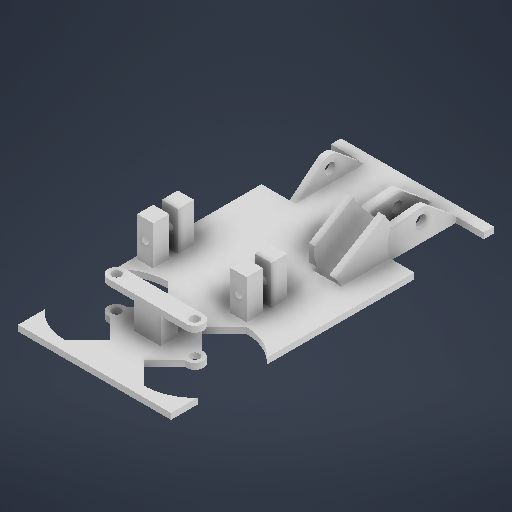
# Autodesk Inventor part: Рама
Saved by Autodesk Inventor 2026.2 (Build 302298000, 298)
## iProperties
Created: 2026-02-19
Part Number: Рама
Material: Типовые
Document SubType Name: Modeling
Designer: Leonid
Density: 1 g/cm^3
Appearance: По умолчанию
Author: Leonid
Autodesk Inventor part; units mm, degrees
ref_plane "XZ Plane" through (0, 0, 0) normal (0, 1, 0) x (-1, 0, 0)
ref_plane "XY Plane" through (0, 0, 0) normal (0, 0, 1) x (1, 0, 0)
sketch "Эскиз1" plane through (0, 0, 0) normal (0, 1, 0) x (-1, 0, 0)
  line L0 (-22.5, -47.5) -> (22.5, -47.5)
  line L1 (22.5, -47.5) -> (22.5, 14.5)
  line L2 (22.5, 47.5) -> (-22.5, 47.5)
  line L3 (-22.5, 47.5) -> (-22.5, 44.5)
  line L4 (-22.5, -47.5) -> (22.5, 47.5) construction
  line L5 (22.5, -47.5) -> (-22.5, 47.5) construction
  line L6 (22.5, 29.5) -> (-22.5, 29.5) construction
  line L7 (-22.5, 44.5) -> (-22.5, 14.5)
  line L8 (-22.5, 14.5) -> (-22.5, -47.5)
  line L9 (22.5, 14.5) -> (22.5, 44.5)
  line L10 (22.5, 44.5) -> (22.5, 47.5)
  circle A0 centre (11.5, 29.5) radius 1.325
  line L11 (22.5, 44.5) -> (5, 44.5)
  line L12 (-22.5, 44.5) -> (-5, 44.5)
  arc A1 (11.5, 27) -> (11.5, 32) centre (11.5, 29.5) ccw
  line L13 (11.5, 32) -> (5, 32)
  circle A2 centre (-11.5, 29.5) radius 1.325
  arc A3 (-11.5, 32) -> (-11.5, 27) centre (-11.5, 29.5) ccw
  line L14 (-11.5, 32) -> (-5, 32)
  line L15 (11.5, 27) -> (-11.5, 27)
  line L16 (22.5, 14.5) -> (-22.5, 14.5)
  line L17 (5, 32) -> (5, 44.5)
  line L18 (-5, 32) -> (-5, 44.5)
  line L19 (-11.5, 44.5) -> (-5, 38)
  line L20 (-11.5, 44.5) -> (-2.3076, 44.5) construction
  line L21 (11.5, 44.5) -> (5, 38)
  line L22 (11.5, 44.5) -> (20.6924, 44.5) construction
  line L23 (5, 38) -> (11, 32)
  line L24 (-5, 38) -> (-11, 32)
  arc A4 (-11.5, 44.5) -> (-22.5, 39.698) centre (-11.5, 29.5) ccw
  arc A5 (22.5, 39.698) -> (11.5, 44.5) centre (11.5, 29.5) ccw
  arc A6 (-22.5, 19.302) -> (-11.5, 14.5) centre (-11.5, 29.5) ccw
  arc A7 (11.5, 14.5) -> (22.5, 19.302) centre (11.5, 29.5) ccw
  line L25 (-11.5, 44.5) -> (-11.5, 14.5) construction
  line L26 (11.5, 44.5) -> (11.5, 14.5) construction
  line L27 (-11, 27) -> (-5, 21)
  line L28 (-11, 27) -> (-2.5147, 27) construction
  line L29 (-5, 21) -> (-11.5, 14.5)
  line L30 (11.5, 14.5) -> (5, 21)
  line L31 (11.5, 14.5) -> (20.6924, 14.5) construction
  line L32 (5, 21) -> (11, 27)
  line L33 (-5.8, 8.55) -> (-10.55, 8.55)
  line L34 (-10.55, 8.55) -> (-10.55, 13.3)
  line L35 (-10.55, 13.3) -> (-5.8, 13.3)
  line L36 (-5.8, 13.3) -> (-5.8, 8.55)
  line L37 (16.95, 8.55) -> (21.7, 8.55)
  line L38 (21.7, 8.55) -> (21.7, 13.3)
  line L39 (21.7, 13.3) -> (16.95, 13.3)
  line L40 (16.95, 13.3) -> (16.95, 8.55)
  line L41 (-5.8, 1.3) -> (-10.55, 1.3)
  line L42 (-10.55, 1.3) -> (-10.55, 6.05)
  line L43 (-10.55, 6.05) -> (-5.8, 6.05)
  line L44 (-5.8, 6.05) -> (-5.8, 1.3)
  line L45 (16.95, 1.3) -> (21.7, 1.3)
  line L46 (21.7, 1.3) -> (21.7, 6.05)
  line L47 (21.7, 6.05) -> (16.95, 6.05)
  line L48 (16.95, 6.05) -> (16.95, 1.3)
  line L49 (22.5, -44.5) -> (-22.5, -44.5)
  line L50 (-22.5, -24.104) -> (-14.25, -24.104)
  line L51 (-14.25, -24.104) -> (-14.25, -44.5)
  line L52 (22.5, -24.104) -> (14.25, -24.104)
  line L53 (14.25, -24.104) -> (14.25, -44.5)
  line L54 (-12.5, -25.63) -> (-7, -25.63)
  line L55 (-7, -25.63) -> (-7, -42.974)
  line L56 (-7, -42.974) -> (-12.5, -42.974)
  line L57 (-12.5, -42.974) -> (-12.5, -25.63)
  line L58 (-12.5, -34.302) -> (-14.25, -34.302) construction
  line L59 (-7.8, 13.3) -> (16.95, 13.3)
  line L60 (16.95, 13.3) -> (16.95, -11.2)
  line L61 (16.95, -11.2) -> (-7.8, -11.2)
  line L62 (-7.8, -11.2) -> (-7.8, 13.3)
  line L63 (-4, 27) -> (4, 27)
  line L64 (4, 27) -> (4, 32)
  line L65 (4, 32) -> (-4, 32)
  line L66 (-4, 32) -> (-4, 27)
  line L67 (-4, 27) -> (4, 32) construction
  line L68 (4, 27) -> (-4, 32) construction
  point P0 (0, 0)
  point P1 (13.75, 44.5)
  point P2 (-12.5, -44.5)
  point P3 (-7.8, 1.3)
  point P4 (16.95, 1.3)
  point P5 (-7.8, 8.55)
  point P6 (-7.8, 6.05)
  point P7 (0, 29.5)
  point P8 (-4, 27)
  point P9 (4, 27)
  dimension "d0" = 45
  dimension "d6" = 3
  dimension "d7" = 2.65
  dimension "d8" = 11
  dimension "d14" = 2.65
  dimension "d15" = 11
  dimension "d16" = 2.5
  dimension "d19" = 10
  dimension "d20" = 12.5
  dimension "d22" = 95
  dimension "d23" = 12.5
  dimension "d25" = 23
  dimension "d26" = 45
  dimension "d27" = 135
  dimension "d29" = 23
  dimension "d30" = 45
  dimension "d31" = 135
  dimension "d37" = 0.5
  dimension "d38" = 32.25
  dimension "d39" = 22.75
  dimension "d40" = 4.75
  dimension "d42" = 5.95
  dimension "d43" = 32.25
  dimension "d44" = 22.75
  dimension "d45" = 4.75
  dimension "d46" = 2.5
  dimension "d60" = 20.3961
  dimension "d61" = 3
  dimension "d62" = 20.396
  dimension "d63" = 8.25
  dimension "d70" = 5.55
  dimension "d71" = 1.75
  dimension "d72" = 5.5
  dimension "d73" = 17.344
  dimension "d101" = 24.5
  dimension "d102" = 2
  dimension "d120" = 8
  constraints: 138 end point, 31 point on line, 23 perpendicular, 22 parallel, 17 horizontal, 12 point on circle, 11 equal length, 10 midpoint, 8 centre point, 6 coincident, 6 collinear, 6 tangent, 1 vertical
  measures "d0" distance of L2.end L2.start
  measures "d6" distance of L9.end L2.start
  measures "d7" diameter of A0
  measures "d8" distance from line of A0.centre L9
  measures "d14" diameter of A2
  measures "d15" distance from line of L7 A2.centre
  measures "d16" radius of A3
  measures "d19" distance between parallel lines of L18 L17
  measures "d20" distance between parallel lines of L16 L15
  measures "d22" distance between parallel lines of L0 L2
  measures "d23" vertical distance of L3.end L14.start
  measures "d25" distance of A2.centre A0.centre
  measures "d26" angle of L19 L20
  measures "d27" angle of L21 L22
  measures "d29" distance of L19.start L21.start
  measures "d30" angle of L27 L28
  measures "d31" angle of L31 L30
  measures "d37" distance of L15.start L32.end
  measures "d38" distance between parallel lines of L34 L38
  measures "d39" distance between parallel lines of L36 L40
  measures "d40" distance between parallel lines of L35 L33
  measures "d42" distance from line of L25.end L33
  measures "d43" distance between parallel lines of L42 L46
  measures "d44" distance between parallel lines of L44 L48
  measures "d45" distance between parallel lines of L43 L41
  measures "d46" distance between parallel lines of L33 L43
  measures "d60" distance of A6.start A4.end
  measures "d61" distance between parallel lines of L0 L49
  measures "d62" distance of L49.end L50.start
  measures "d63" distance of L50.start L50.end
  measures "d70" distance between parallel lines of L1 L40
  measures "d71" distance between parallel lines of L51 L57
  measures "d72" distance between parallel lines of L57 L55
  measures "d73" distance between parallel lines of L56 L54
  measures "d101" distance between parallel lines of L59 L61
  measures "d102" distance between parallel lines of L44 L62
  measures "d120" distance between parallel lines of L64 L66
extrude "Выдавливание1" add sketch "Эскиз1" along normal blind 1.75 contours L8 L49 L1 L0 | L8 L16 L1 L52 L53 L49 L51 L50 | L7 A6 L16 | L16 A7 L9 | L29 L27 L15 L32 L30 L16 | L7 L12 A4 | A5 L11 L9 | L3 L2 L10 L11 L17 L13 A1 L15 L64 L65 L66 A3 L14 L18 L12 | L12 L18 L19 | L21 L17 L11 | L18 L14 L24 | L66 L65 L64 L15 | L23 L13 L17 | L36 L59 L40 L60 L48 L61 L62 L41 L44 L43 L33 | L33 L62 L35 L36 | L33 L34 L35 L62 | L62 L41 L42 L43 | L43 L44 L41 L62 | L39 L38 L37 L40 | L47 L46 L45 L48
extrude "Выдавливание3" add sketch "Эскиз1" along normal blind 13.25 contours L33 L62 L35 L36 | L33 L34 L35 L62 | L62 L41 L42 L43 | L43 L44 L41 L62 | L39 L38 L37 L40 | L47 L46 L45 L48
sketch "Эскиз3" plane through (10.55, 1.75, 1.3) normal (0, 0, -1) x (-1, 0, 0)
  line L0 (-11.95, 0) -> (33.05, 0) projected
  line L1 (0, 0) -> (0, 11.5) projected
  point P0 (10.55, -1.75)
  point P1 (2.375, 5.95)
  point P2 (29.875, 5.95)
  dimension "d49" = 27.5
  dimension "d50" = 5.95
  dimension "d51" = 2.375
  dimension "d52" = 5.95
  measures "d49" distance of point (29.875, 5.95) point (2.375, 5.95)
  measures "d50" distance from line of L0 point (2.375, 5.95)
  measures "d51" distance from line of L1 point (2.375, 5.95)
  measures "d52" distance from line of L0 point (29.875, 5.95)
hole "Отверстие1" at (8.175, 7.7, 1.3) at (-19.325, 7.7, 1.3) direction (0, 0, 1) diameter 2.1 end through all
sketch "Эскиз4" plane through (14.25, 0, -24.104) normal (1, 0, 0) x (0, 0, -1)
  line L0 (0, 1.75) -> (20.396, 1.75) projected
  circle A0 centre (10.198, 5.6) radius 1.575
  line L1 (10.198, 5.6) -> (10.198, 1.75) construction
  arc A1 (12.4201, 8.3041) -> (7.9759, 8.3041) centre (10.198, 5.6) ccw
  line L2 (0, 1.75) -> (7.9759, 8.3041)
  line L3 (12.4201, 8.3041) -> (20.396, 1.75)
  point P0 (-24.104, 0)
  dimension "d64" = 3.15
  dimension "d65" = 3.85
  dimension "d66" = 3.5
  constraints: 6 end point, 2 centre point, 2 point on circle, 2 tangent, 1 coincident, 1 midpoint, 1 vertical
  measures "d64" diameter of A0
  measures "d65" distance of L1.start L1.end
  measures "d66" radius of A1
extrude "Выдавливание4" add sketch "Эскиз4" against normal blind 1.75
mirror "Зеркальное отражение1" about plane through (0, 0, 0) normal (1, 0, 0) of "Выдавливание4"
ref_plane "РабПлоскость2" through (9.85, 0, 0) normal (1, 0, 0) x (0, 1, 0)
sketch "Эскиз5" plane through (9.85, 0, 0) normal (1, 0, 0) x (0, 1, 0)
  circle A0 centre (5.6, -34.302) radius 1.575 projected
  line L0 (5.6, -34.302) -> (5.6, -24.814)
  line L1 (1.75, -24.104) -> (1.75, -25.63) projected
  arc A1 (14.3322, -38.0128) -> (5.6, -24.814) centre (5.6, -34.302) ccw
  line L2 (6.8478, -6.6784) -> (15.6371, -21.2299)
  line L3 (15.6371, -21.2299) -> (8.7893, -25.3661)
  line L4 (8.7893, -25.3661) -> (0, -10.8145)
  line L5 (0, -10.8145) -> (6.8478, -6.6784)
  line L6 (16.0736, -20.9662) -> (8.3528, -25.6297)
  line L7 (8.3528, -25.6297) -> (14.557, -35.9014)
  line L8 (14.557, -35.9014) -> (22.2779, -31.2379)
  line L9 (22.2779, -31.2379) -> (16.0736, -20.9662)
  line L10 (22.2779, -31.2379) -> (8.3528, -25.6297) construction
  line L11 (5.6, -34.302) -> (19.1758, -26.1021) construction
  line L12 (0, 19.302) -> (0, -24.104) projected
  line L13 (13.4972, -22.5225) -> (4.7079, -7.9709)
  line L14 (1.75, 30.825) -> (1.75, 28.175) projected
  line L15 (1.75, 30.825) -> (1.75, 28.175) projected
  line L16 (1.75, 13.3) -> (1.75, 8.55) projected
  line L17 (1.75, 8.55) -> (1.75, 13.3) projected
  line L18 (1.75, 8.55) -> (1.75, 13.3) projected
  line L19 (1.75, 13.3) -> (1.75, 8.55) projected
  line L20 (1.75, 1.3) -> (1.75, 6.05) projected
  line L21 (1.75, 6.05) -> (1.75, 1.3) projected
  line L22 (1.75, 1.3) -> (1.75, 6.05) projected
  line L23 (1.75, 6.05) -> (1.75, 1.3) projected
  line L24 (1.75, -44.5) -> (1.75, -24.104) projected
  line L25 (1.75, -24.104) -> (1.75, 19.302) projected
  line L26 (1.75, 19.302) -> (1.75, 14.5) projected
  line L27 (1.75, 14.5) -> (1.75, 21) projected
  line L28 (1.75, 21) -> (1.75, 27) projected
  line L29 (1.75, 27) -> (1.75, 32) projected
  line L30 (1.75, 32) -> (1.75, 38) projected
  line L31 (1.75, 38) -> (1.75, 44.5) projected
  line L32 (1.75, 44.5) -> (1.75, 39.698) projected
  line L33 (1.75, 39.698) -> (1.75, 47.5) projected
  line L34 (1.75, 47.5) -> (1.75, 39.698) projected
  line L35 (1.75, 39.698) -> (1.75, 44.5) projected
  line L36 (1.75, 44.5) -> (1.75, 38) projected
  line L37 (1.75, 38) -> (1.75, 32) projected
  line L38 (1.75, 32) -> (1.75, 27) projected
  line L39 (1.75, 27) -> (1.75, 21) projected
  line L40 (1.75, 21) -> (1.75, 14.5) projected
  line L41 (1.75, 14.5) -> (1.75, 19.302) projected
  line L42 (1.75, 19.302) -> (1.75, -24.104) projected
  line L43 (1.75, -24.104) -> (1.75, -25.63) projected
  line L44 (1.75, -25.63) -> (1.75, -42.974) projected
  line L45 (1.75, -42.974) -> (1.75, -44.5) projected
  line L46 (1.75, -44.5) -> (1.75, -47.5) projected
  line L47 (1.75, -47.5) -> (1.75, -44.5) projected
  line L48 (8.3041, -32.0799) -> (1.75, -24.104) projected
  line L49 (0, -24.104) -> (1.75, -24.104) projected
  arc A2 (10.2878, -24.461) -> (7.7295, -23.6115) centre (5.6, -34.302) ccw
  arc A3 (7.7295, -23.6115) -> (1.75, -24.104) centre (5.6, -34.302) ccw
  line L50 (9.0866, -33.9962) -> (8.3528, -25.6297)
  arc A4 (8.3041, -36.5241) -> (8.3041, -32.0799) centre (5.6, -34.302) ccw projected
  arc A5 (5.6, -24.814) -> (1.75, -25.6302) centre (5.6, -34.302) ccw
  line L51 (8.3041, -36.5241) -> (1.75, -44.5) projected
  point P0 (0, 0)
  point P1 (12.2132, -23.298)
  point P2 (15.3153, -28.4338)
  point P3 (1.75, -9.7575)
  point P4 (13.4972, -22.5225)
  point P5 (11.5647, -26.9233)
  point P6 (14.9935, -35.6378)
  point P7 (5.6, -28.7892)
  point P8 (1.75, -25.6302)
  point P9 (2.7052, -25.2664)
  point P10 (1.75, -25.63)
  dimension "d76" = 8
  dimension "d77" = 17
  dimension "d78" = 11.35
  dimension "d79" = 12
  dimension "d80" = 9.02
  dimension "d81" = 5.5
  constraints: 26 end point, 10 point on circle, 7 perpendicular, 7 point on line, 4 centre point, 4 midpoint, 3 coincident, 1 collinear, 1 tangent, 1 vertical
  measures "d76" distance of L4.end L2.start
  measures "d77" distance between parallel lines of L3 L5
  measures "d78" distance of L0.start point (15.315, -28.434)
  measures "d79" distance between parallel lines of L3 L8
  measures "d80" distance of L7.end L8.end
  measures "d81" distance between parallel lines of L4 L13
extrude "Выдавливание5" add sketch "Эскиз5" along normal blind 5.5 contours L25 L4 A3 | A2 L4 L25 L5 L13 L3
extrude "Выдавливание6" add sketch "Эскиз5" along normal blind 4.4 contours L48 A5 L0 | L0 A1 L6 L50 A4 L48 | A5 L48 A3 L4 A1 | A5 L1 L48 | L4 A2 L3
extrude "Выдавливание8" add sketch "Эскиз5" against normal blind 5.5 contours A5 L48 A3 L4 A1 | A5 L1 L48 | L4 A2 L3 | L25 L4 A3 | A2 L4 L25 L5 L13 L3
extrude "Выдавливание9" add sketch "Эскиз5" against normal blind 5.5 contours L48 A5 L0 | L0 A1 L6 L50 A4 L48 | L48 A4 L51 L24 A5
extrude "Выдавливание7" cut sketch "Эскиз5" along normal mid plane 5.3 contours L48 A5 L0 | L0 A1 L6 L50 A4 L48 | L48 A4 L51 L24 A5
extrude "Выдавливание10" cut sketch "Эскиз1" along normal blind 10.15 contours L36 L59 L40 L60 L48 L61 L62 L41 L44 L43 L33
extrude "Выдавливание11" add sketch "Эскиз1" along normal blind 1.75 contours L36 L59 L40 L60 L48 L61 L62 L41 L44 L43 L33
sketch "Эскиз6" plane through (15.35, 10.2878, -24.461) normal (0, 0.517018, -0.8559746) x (-1, 0, 0)
  line L0 (11, 3.7494) -> (0, 3.7494) projected
  line L1 (2.85, -1.7506) -> (8.15, -1.7506) projected
  line L2 (5.5, 2.2494) -> (5.5, -1.7506)
  point P0 (15.35, 3.8406)
  dimension "d100" = 4
  constraints: 2 end point, 1 midpoint, 1 vertical
  measures "d100" distance of L2.start L2.end
hole "Отверстие2" at (9.85, 12.2132, -23.298) direction (0, -0.517018, 0.8559746) diameter 8 depth 17
extrude "Выдавливание12" add sketch "Эскиз1" along normal blind 9.45 contours L66 L65 L64 L15
ref_plane "РабПлоскость4" through (-22.5, 0, 17.8) normal (0, 0, 1) x (1, 0, 0)
sketch "Эскиз7" plane through (-22.5, 0, 17.8) normal (0, 0, 1) x (1, 0, 0)
  circle A0 centre (22.5, 8) radius 7
  line L0 (0, 1.75) -> (45, 1.75) projected
  line L1 (22.5, 1.75) -> (22.5, 8) construction
  point P0 (22.5, 0)
  point P1 (25.6524, 1.75)
  point P2 (19.3476, 1.75)
  dimension "d110" = 14
  dimension "d111" = 6.25
  constraints: 2 end point, 1 centre point, 1 midpoint, 1 vertical
  measures "d110" diameter of A0
  measures "d111" distance of L1.start L1.end
extrude "Выдавливание15" cut sketch "Эскиз7" along normal blind 8.75 contours L0 A0 picked at (21.9599, 1.5634)
sketch "Эскиз8" plane through (0, 9.45, 0) normal (0, 1, 0) x (1, 0, 0)
  arc A0 (11.5, -32) -> (11.5, -27) centre (11.5, -29.5) ccw projected
  line L0 (-11.5, -27) -> (11.5, -27) projected
  arc A1 (-11.5, -27) -> (-11.5, -32) centre (-11.5, -29.5) ccw projected
  line L1 (-11.5, -32) -> (-11, -32) construction
  line L2 (-11.5, -32) -> (11.5, -32)
  circle A2 centre (-11.5, -29.5) radius 1.325 projected
  circle A3 centre (11.5, -29.5) radius 1.325 projected
  point P0 (0, 0)
  constraints: 2 end point, 1 horizontal, 1 tangent
extrude "Выдавливание16" add sketch "Эскиз8" along normal blind 1.75
